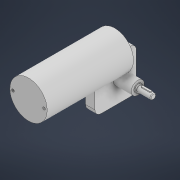
# Autodesk Inventor part: motor
Saved by Autodesk Inventor 2021 (Build 250183000, 183)
## iProperties
Created: 2021-06-20
Part Number: motor
Material: Generic
Document SubType Name: Modeling
Designer: Watchdog
Density: 1 g/cm^3
Appearance: Default
Author: Watchdog
Autodesk Inventor part; units mm, degrees
ref_plane "XY Plane" through (0, 0, 0) normal (0, 0, 1) x (1, 0, 0)
sketch "Sketch1" plane through (0, 0, 0) normal (0, 0, 1) x (1, 0, 0)
  circle A0 centre (0, 0) radius 30
  dimension "d0" = 60
  constraints: 1 centre point, 1 coincident
  measures "d0" diameter of A0
extrude "Extrusion1" add sketch "Sketch1" along normal blind 139
ref_plane "Work Plane1" through (62, 0, 0) normal (1, 0, 0) x (0, 1, 0)
ref_plane "Work Plane2" through (0, 0, 0) normal (1, 0, 0) x (0, 1, 0)
sketch "Sketch2" plane through (0, 0, 0) normal (1, 0, 0) x (0, 1, 0)
  point P0 (0, 0)
ref_plane "Work Plane3" through (0, 0, 0) normal (0, 0, -1) x (-1, 0, 0)
sketch "Sketch3" plane through (0, 0, 0) normal (0, 0, -1) x (-1, 0, 0)
  line L0 (0, -34.6) -> (-62, -34.6)
  line L1 (-62, -34.6) -> (-62, -30.1)
  line L2 (-62, -30.1) -> (-40, -30.1)
  line L3 (-40, -30.1) -> (-40, -29.1)
  line L4 (-40, -29.1) -> (-38, -29.1)
  line L5 (-38, -29.1) -> (-38, -28.1)
  line L6 (-38, -28.1) -> (-37, -28.1)
  line L7 (-37, -28.1) -> (-37, -24.1)
  line L8 (-37, -24.1) -> (0, -24.1)
  line L9 (0, -24.1) -> (0, -34.6)
  point P0 (0, 0)
  dimension "d6" = 62
  dimension "d7" = 34.6
  dimension "d15" = 4.5
  dimension "d16" = 22
  dimension "d17" = 1
  dimension "d18" = 2
  dimension "d19" = 1
  dimension "d20" = 1
  dimension "d21" = 4
  dimension "d22" = 0
  constraints: 20 end point, 6 perpendicular, 3 vertical, 1 horizontal
  measures "d6" distance of L0.start L0.end
  measures "d7" distance from line of point (0, 0) L0
  measures "d15" distance of L0.end L1.end
  measures "d16" distance of L1.end L2.end
  measures "d17" distance of L2.end L3.end
  measures "d18" distance of L3.end L4.end
  measures "d19" distance of L4.end L5.end
  measures "d20" distance of L5.end L6.end
  measures "d21" distance of L6.end L7.end
  measures "d22" distance from line of point (0, 0) L9
sketch "Sketch4" plane through (0, 0, 0) normal (1, 0, 0) x (0, 1, 0)
  line L0 (-30, 0) -> (-30, 139) projected
  line L1 (0, 39.5) -> (-70.6, 39.5)
  line L2 (-70.6, -27) -> (0, -27)
  line L3 (0, -27) -> (0, 39.5)
  line L4 (-70.6, 39.5) -> (-70.6, -27)
  line L5 (30, 0) -> (30, 139) projected
  point P0 (0, 0)
  point P1 (-30, 39.5)
  dimension "d11" = 0
  dimension "d12" = 99.5
  dimension "d13" = 66.5
  dimension "d14" = 100.6
  constraints: 8 end point, 1 horizontal, 1 parallel, 1 vertical
  measures "d11" distance from line of point (0, 0) L3
  measures "d12" distance from line of L1 point (-30, 139)
  measures "d13" distance between parallel lines of L1 L2
  measures "d14" distance between parallel lines of L4 L5
extrude "Extrusion2" add sketch "Sketch4" along normal mid plane 15
revolve "Revolution1" add sketch "Sketch3" angle 360 about axis through (0, -34.6, 0) along (1, 0, 0)
ref_plane "Work Plane4" through (51, -30.1, 0) normal (0, 1, 0) x (-1, 0, 0)
sketch "Sketch5" plane through (51, -30.1, 0) normal (0, 1, 0) x (-1, 0, 0)
  line L0 (-11, -4.5) -> (-11, 4.5) projected
  line L1 (99.4, 0) -> (-29.4, 0) projected
  line L2 (6.5, 0) -> (-6.5, 0) construction
  line L3 (6.5, 1.5) -> (-6.5, 1.5)
  line L4 (-6.5, -1.5) -> (6.5, -1.5)
  arc A0 (6.5, -1.5) -> (6.5, 1.5) centre (6.5, 0) ccw
  arc A1 (-6.5, 1.5) -> (-6.5, -1.5) centre (-6.5, 0) ccw
  point P0 (51, 0)
  point P1 (0, 0)
  dimension "d28" = 3
  dimension "d29" = 0
  dimension "d30" = 13
  dimension "d31" = 4.5
  constraints: 8 end point, 4 point on circle, 4 tangent, 2 centre point, 1 horizontal, 1 midpoint, 1 parallel
  measures "d28" distance between parallel lines of L4 L3
  measures "d29" distance from line of L1 point (0, 0)
  measures "d30" distance of L2.end L2.start
  measures "d31" distance from line of L0 L2.end
extrude "Extrusion3" add sketch "Sketch5" against normal up to surface round surface about axis through (51, -34.6, 0) along (-1, 0, 0) radius 4.5 far side no
sketch "Sketch6" plane through (51, -30.1, 0) normal (0, 1, 0) x (1, 0, 0)
  arc A0 (-8, 0) -> (-6.5, -1.5) centre (-6.5, 0) ccw projected
  line L0 (-6.5, -1.5) -> (6.5, -1.5) projected
  arc A1 (6.5, -1.5) -> (8, 0) centre (6.5, 0) ccw projected
  arc A2 (8, 0) -> (6.5, 1.5) centre (6.5, 0) ccw projected
  line L1 (6.5, 1.5) -> (-6.5, 1.5) projected
  arc A3 (-6.5, 1.5) -> (-8, 0) centre (-6.5, 0) ccw projected
  point P0 (-51, 0)
extrude "Extrusion4" add sketch "Sketch6" along normal blind 1.3
chamfer "Chamfer1" distance 1 angle 45 1 edges at (62, -39.1, 0)
fillet "Fillet1" radius 10 3 edges at (0, 0, -27) (0, -70.6, -27) (0, -70.6, 39.5)
sketch "Sketch7" plane through (0, 0, 139) normal (0, 0, 1) x (1, 0, 0)
  point P0 (0, 0)
  point P1 (0, 0)
  point P2 (-25, 0)
  point P3 (25, 0)
  dimension "d42" = 0
  dimension "d43" = 0
  dimension "d44" = 25
  dimension "d45" = 25
  measures "d42" vertical distance of point (0, 0) point (25, 0)
  measures "d43" vertical distance of point (0, 0) point (-25, 0)
  measures "d44" distance of point (0, 0) point (-25, 0)
  measures "d45" distance of point (0, 0) point (25, 0)
hole "Hole1" at (-25, 0, 139) at (25, 0, 139) direction (0, 0, -1) diameter 4.134 depth 8 tip angle 118 thread size "M5x0.8" class "6H" standard "ISO Metric profile"
body "Solid1"
